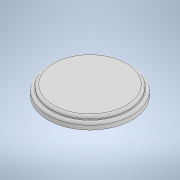
# Autodesk Inventor part: Chess Piece Base
Saved by Autodesk Inventor 2022 (Build 260153000, 153)
## iProperties
Created: 2022-04-22
Part Number: Chess Piece Base
Material: Generic
Document SubType Name: Modeling
Designer: Nick
Density: 1 g/cm^3
Appearance: Default
Author: Nick
Autodesk Inventor part; units mm, degrees
ref_plane "YZ Plane" through (0, 0, 0) normal (1, 0, 0) x (0, 1, 0)
ref_plane "XZ Plane" through (0, 0, 0) normal (0, 1, 0) x (-1, 0, 0)
ref_plane "XY Plane" through (0, 0, 0) normal (0, 0, 1) x (1, 0, 0)
sketch "Sketch1" plane through (0, 0, 0) normal (0, 0, 1) x (1, 0, 0)
  line L0 (0, 0) -> (0, 19.8394)
  line L1 (0, 0) -> (12.7, 0)
  line L2 (12.7, 0) -> (12.7, 2)
  line L3 (12.7, 2) -> (11.7, 2)
  line L4 (11.7, 2) -> (11.7, 3)
  line L5 (11.7, 3) -> (0, 3)
  dimension "d0" = 12.7
  dimension "d1" = 2
  dimension "d2" = 1
  dimension "d3" = 1
  constraints: 12 end point, 4 perpendicular, 1 horizontal, 1 point on line, 1 vertical
  measures "d0" distance between parallel lines of L0 L2
  measures "d1" distance of L1.end L2.end
  measures "d2" distance of L3.end L4.end
  measures "d3" distance of L2.end L3.end
revolve "Revolution1" add sketch "Sketch1" angle 360 about axis through (0, 0, 0) along (0, 1, 0)
fillet "Fillet1" radius 0.75 2 edges at (-12.7, 2, 0) (-11.7, 3, 0)
body "Solid1"
